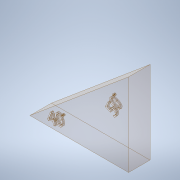
# Autodesk Inventor part: 40-50-4in-Template
Saved by Autodesk Inventor 2020.2 (Build 242310000, 310)
## iProperties
Created: 2020-01-27
Part Number: 40-50-4in-Template
Material: PET Plastic
Document SubType Name: Modeling
Designer: robst
Density: 1.541 g/cm^3
Appearance: Polycarbonate - Smoked
Author: robst
Autodesk Inventor part; units mm, degrees
ref_plane "YZ Plane" through (0, 0, 0) normal (1, 0, 0) x (0, 1, 0)
ref_plane "XZ Plane" through (0, 0, 0) normal (0, 1, 0) x (-1, 0, 0)
ref_plane "XY Plane" through (0, 0, 0) normal (0, 0, 1) x (1, 0, 0)
sketch "Sketch1" plane through (0, 0, 0) normal (0, 0, 1) x (1, 0, 0)
  line L0 (0, 0) -> (116.7452, 97.9608)
  line L1 (0, 0) -> (152.4, 0) construction
  line L2 (116.7452, 97.9608) -> (116.7452, 0)
  line L3 (116.7452, 0) -> (0, 0)
  dimension "d0" = 152.4
  dimension "d1" = 40
  constraints: 8 end point, 1 equal length, 1 horizontal, 1 perpendicular, 1 vertical
  measures "d0" distance of L0.start L0.end
  measures "d1" angle of L1 L0
extrude "Extrusion1" add sketch "Sketch1" along normal mid plane 25.4
sketch "Sketch2" plane through (0, 0, 12.7) normal (0, 0, 1) x (1, 0, 0)
  line L0 (0, 0) -> (116.7452, 0) construction
  line L1 (0, 0) -> (116.7452, 42.4918) construction
  line L2 (116.7452, 0) -> (116.7452, 97.9608) construction
  line L3 (29.7312, 8.7075) -> (28.3096, 8.1901)
  line L4 (28.3096, 8.1901) -> (29.8021, 4.0895)
  line L5 (29.8021, 4.0895) -> (28.2644, 3.5299)
  line L6 (28.2644, 3.5299) -> (26.7719, 7.6304)
  line L7 (26.7719, 7.6304) -> (21.5012, 5.712)
  line L8 (21.5012, 5.712) -> (20.8887, 7.3948)
  line L9 (20.8887, 7.3948) -> (23.9884, 15.4886)
  line L10 (23.9884, 15.4886) -> (25.4584, 16.0236)
  line L11 (25.4584, 16.0236) -> (27.8414, 9.4763)
  line L12 (27.8414, 9.4763) -> (29.2631, 9.9938)
  line L13 (29.2631, 9.9938) -> (29.7312, 8.7075)
  line L14 (26.3037, 8.9166) -> (24.6071, 13.5781)
  line L15 (24.6071, 13.5781) -> (22.2902, 7.4559)
  line L16 (22.2902, 7.4559) -> (26.3037, 8.9166)
  spline S0 degree 2 poles (37.7558, 13.742) (38.9245, 10.5312) (38.1527, 6.8442) (36.2088, 6.1366) knots 0 0 0 1 2 2 2
  spline S1 degree 2 poles (36.2088, 6.1366) (34.2359, 5.4186) (31.2729, 7.812) (30.1289, 10.9551) knots 0 0 0 1 2 2 2
  spline S2 degree 2 poles (30.1289, 10.9551) (28.9532, 14.1852) (29.7321, 17.8529) (31.6856, 18.564) knots 0 0 0 1 2 2 2
  spline S3 degree 2 poles (31.6856, 18.564) (33.6488, 19.2785) (36.6224, 16.8561) (37.7558, 13.742) knots 0 0 0 1 2 2 2
  spline S4 degree 2 poles (37.0291, 9.3594) (37.0465, 10.0339) (36.5781, 11.9224) (36.1311, 13.1506) knots 0 0 0 1 2 2 2
  spline S5 degree 2 poles (36.1311, 13.1506) (35.6841, 14.3789) (34.8324, 16.117) (34.3689, 16.6382) knots 0 0 0 1 2 2 2
  spline S6 degree 2 poles (34.3689, 16.6382) (33.9053, 17.1595) (32.8352, 17.4819) (32.1679, 17.239) knots 0 0 0 1 2 2 2
  spline S7 degree 2 poles (32.1679, 17.239) (31.5005, 16.9961) (30.8686, 16.0542) (30.846, 15.3341) knots 0 0 0 1 2 2 2
  spline S8 degree 2 poles (30.846, 15.3341) (30.826, 14.6368) (31.3277, 12.7166) (31.7536, 11.5464) knots 0 0 0 1 2 2 2
  spline S9 degree 2 poles (31.7536, 11.5464) (32.2112, 10.2892) (32.9784, 8.6627) (33.4692, 8.0966) knots 0 0 0 1 2 2 2
  spline S10 degree 2 poles (33.4692, 8.0966) (33.9266, 7.5622) (35.0302, 7.2081) (35.7266, 7.4616) knots 0 0 0 1 2 2 2
  spline S11 degree 2 poles (35.7266, 7.4616) (36.3842, 7.7009) (37.0161, 8.6428) (37.0291, 9.3594) knots 0 0 0 1 2 2 2
  spline S12 degree 2 poles (38.4763, 17.6439) (37.9694, 17.4594) (36.9953, 17.9137) (36.815, 18.409) knots 0 0 0 1 2 2 2
  spline S13 degree 2 poles (36.815, 18.409) (36.6305, 18.9159) (37.0848, 19.89) (37.5916, 20.0745) knots 0 0 0 1 2 2 2
  spline S14 degree 2 poles (37.5916, 20.0745) (38.087, 20.2548) (39.0611, 19.8005) (39.2456, 19.2937) knots 0 0 0 1 2 2 2
  spline S15 degree 2 poles (39.2456, 19.2937) (39.4259, 18.7983) (38.9716, 17.8242) (38.4763, 17.6439) knots 0 0 0 1 2 2 2
  spline S16 degree 2 poles (37.9564, 19.0723) (37.7375, 18.9926) (37.8172, 18.7738) knots 0 0 0 1 1 1
  spline S17 degree 2 poles (37.8172, 18.7738) (37.8926, 18.5664) (38.1115, 18.6461) knots 0 0 0 1 1 1
  spline S18 degree 2 poles (38.1115, 18.6461) (38.3189, 18.7216) (38.2434, 18.9289) knots 0 0 0 1 1 1
  spline S19 degree 2 poles (38.2434, 18.9289) (38.1637, 19.1478) (37.9564, 19.0723) knots 0 0 0 1 1 1
  dimension "d4" = 20
  constraints: 2 end point, 1 point on line, 1 other
  measures "d4" angle of L1 L0
sketch "Sketch3" plane through (0, 0, 12.7) normal (0, 0, 1) x (1, 0, 0)
  line L0 (116.7452, 97.9608) -> (0, 0) construction
  line L1 (116.7452, 97.9608) -> (71.0653, 0) construction
  line L2 (0, 0) -> (116.7452, 0) construction
  line L3 (116.7452, 0) -> (116.7452, 97.9608) construction
  spline S0 degree 2 poles (99.861, 56.2734) (100.6912, 55.8863) (101.861, 54.6935) (102.1572, 53.9649) knots 0 0 0 1 2 2 2
  spline S1 degree 2 poles (102.1572, 53.9649) (102.4534, 53.2363) (102.3855, 51.5079) (101.9679, 50.6124) knots 0 0 0 1 2 2 2
  spline S2 degree 2 poles (101.9679, 50.6124) (101.5852, 49.7916) (100.4733, 48.3569) (99.9101, 47.9041) knots 0 0 0 1 2 2 2
  line L4 (99.9101, 47.9041) -> (98.2778, 48.6653)
  line L5 (98.2778, 48.6653) -> (98.33, 48.7772)
  spline S3 degree 2 poles (98.33, 48.7772) (98.5433, 48.8935) (99.1879, 49.3992) (99.5241, 49.7307) knots 0 0 0 1 2 2 2
  spline S4 degree 2 poles (99.5241, 49.7307) (99.8958, 50.1138) (100.4253, 50.7867) (100.6472, 51.2624) knots 0 0 0 1 2 2 2
  spline S5 degree 2 poles (100.6472, 51.2624) (100.8646, 51.7288) (100.9377, 52.7621) (100.7218, 53.2489) knots 0 0 0 1 2 2 2
  spline S6 degree 2 poles (100.7218, 53.2489) (100.5115, 53.699) (99.7366, 54.4237) (99.121, 54.7108) knots 0 0 0 1 2 2 2
  spline S7 degree 2 poles (99.121, 54.7108) (98.5054, 54.9978) (97.5653, 55.0274) (97.1563, 54.832) knots 0 0 0 1 2 2 2
  spline S8 degree 2 poles (97.1563, 54.832) (96.7149, 54.6404) (96.02, 53.7834) (95.746, 53.1958) knots 0 0 0 1 2 2 2
  spline S9 degree 2 poles (95.746, 53.1958) (95.4502, 52.5615) (95.0589, 51.211) (94.9645, 50.7894) knots 0 0 0 1 2 2 2
  line L6 (94.9645, 50.7894) -> (89.0323, 53.5557)
  line L7 (89.0323, 53.5557) -> (91.9769, 59.8704)
  line L8 (91.9769, 59.8704) -> (93.3293, 59.2397)
  line L9 (93.3293, 59.2397) -> (91.0763, 54.4081)
  line L10 (91.0763, 54.4081) -> (94.1451, 52.9771)
  spline S10 degree 2 poles (94.1451, 52.9771) (94.2382, 53.2743) (94.4625, 53.8284) (94.5669, 54.0522) knots 0 0 0 1 2 2 2
  spline S11 degree 2 poles (94.5669, 54.0522) (94.9801, 54.9383) (95.839, 56.0254) (96.5291, 56.385) knots 0 0 0 1 2 2 2
  spline S12 degree 2 poles (96.5291, 56.385) (97.2235, 56.7539) (98.8164, 56.7606) (99.861, 56.2734) knots 0 0 0 1 2 2 2
  spline S13 degree 2 poles (101.877, 66.0759) (104.9737, 64.6318) (107.0351, 61.4789) (106.1608, 59.6041) knots 0 0 0 1 2 2 2
  spline S14 degree 2 poles (106.1608, 59.6041) (105.2735, 57.7013) (101.486, 57.2985) (98.4546, 58.7121) knots 0 0 0 1 2 2 2
  spline S15 degree 2 poles (98.4546, 58.7121) (95.3392, 60.1649) (93.2964, 63.309) (94.175, 65.1932) knots 0 0 0 1 2 2 2
  spline S16 degree 2 poles (94.175, 65.1932) (95.058, 67.0867) (98.8735, 67.4764) (101.877, 66.0759) knots 0 0 0 1 2 2 2
  spline S17 degree 2 poles (104.462, 62.463) (103.9974, 62.9522) (102.3308, 63.9565) (101.1463, 64.5088) knots 0 0 0 1 2 2 2
  spline S18 degree 2 poles (101.1463, 64.5088) (99.9617, 65.0612) (98.1304, 65.688) (97.4341, 65.7289) knots 0 0 0 1 2 2 2
  spline S19 degree 2 poles (97.4341, 65.7289) (96.7377, 65.7697) (95.753, 65.2409) (95.4529, 64.5973) knots 0 0 0 1 2 2 2
  spline S20 degree 2 poles (95.4529, 64.5973) (95.1528, 63.9537) (95.372, 62.8409) (95.8652, 62.3156) knots 0 0 0 1 2 2 2
  spline S21 degree 2 poles (95.8652, 62.3156) (96.3441, 61.8084) (98.0566, 60.8054) (99.1853, 60.2791) knots 0 0 0 1 2 2 2
  spline S22 degree 2 poles (99.1853, 60.2791) (100.3978, 59.7137) (102.0904, 59.1061) (102.8378, 59.0529) knots 0 0 0 1 2 2 2
  spline S23 degree 2 poles (102.8378, 59.0529) (103.5391, 58.9984) (104.5698, 59.5284) (104.883, 60.2) knots 0 0 0 1 2 2 2
  spline S24 degree 2 poles (104.883, 60.2) (105.1787, 60.8343) (104.9596, 61.9471) (104.462, 62.463) knots 0 0 0 1 2 2 2
  spline S25 degree 2 poles (99.6273, 69.3443) (99.3994, 68.8555) (98.3894, 68.4879) (97.9116, 68.7106) knots 0 0 0 1 2 2 2
  spline S26 degree 2 poles (97.9116, 68.7106) (97.4228, 68.9386) (97.0551, 69.9486) (97.2831, 70.4375) knots 0 0 0 1 2 2 2
  spline S27 degree 2 poles (97.2831, 70.4375) (97.5059, 70.9152) (98.5159, 71.2828) (99.0048, 71.0549) knots 0 0 0 1 2 2 2
  spline S28 degree 2 poles (99.0048, 71.0549) (99.4825, 70.8321) (99.8501, 69.8221) (99.6273, 69.3443) knots 0 0 0 1 2 2 2
  spline S29 degree 2 poles (98.2497, 69.9868) (98.1512, 69.7757) (98.3623, 69.6772) knots 0 0 0 1 1 1
  spline S30 degree 2 poles (98.3623, 69.6772) (98.5623, 69.584) (98.6608, 69.7951) knots 0 0 0 1 1 1
  spline S31 degree 2 poles (98.6608, 69.7951) (98.754, 69.995) (98.554, 70.0883) knots 0 0 0 1 1 1
  spline S32 degree 2 poles (98.554, 70.0883) (98.3429, 70.1867) (98.2497, 69.9868) knots 0 0 0 1 1 1
  dimension "d5" = 25
  constraints: 2 end point, 1 point on line, 1 other
  measures "d5" angle of L1 L3
extrude "Extrusion2" cut sketch "Sketch2" against normal blind 2.54
extrude "Extrusion3" cut sketch "Sketch3" against normal blind 2.54
body "Solid1"
